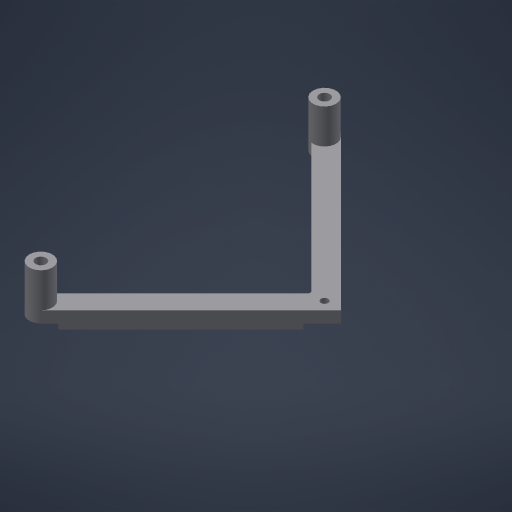
# Autodesk Inventor part: WIDE SCREEN HOLDER 2SCREEN
Saved by Autodesk Inventor 2023.3 (Build 273359000, 359)
## iProperties
RuleStatus: InUse
Created: 2023-07-19
Material: Generic
Catalog Web Link: https://www.janelia.org/
Vendor: HHMI: JRC - jET
Document SubType Name: Modeling
Designer: jagers
Density: 1 g/cm^3
Appearance: Default
Part Number: WIDE SCREEN HOLDER 2SCREEN
AfterDocSave0: file://Part Number Cleaner
DESIGN DEPARTMENT: HHMI: JRC - jET
ALTERED ITEM PART NUMBER: N/A
ALTERED ITEM VENDOR: N/A
ALTERED ITEM DESCRIPTION: N/A
Title: Standard
Author: jagers
Revision Number: 0
Autodesk Inventor part; units mm, degrees
ref_plane "YZ Plane" through (0, 0, 0) normal (1, 0, 0) x (0, 1, 0)
ref_plane "XZ Plane" through (0, 0, 0) normal (0, 1, 0) x (-1, 0, 0)
sketch "Sketch1" plane through (0, 0, 0) normal (0, 1, 0) x (-1, 0, 0)
  line L0 (-41.3092, 0) -> (0, 41.3092)
  circle A0 centre (-36.8191, 0) radius 1.016
  arc A1 (-32.8821, 0) -> (-34.0352, 2.7839) centre (-36.8191, 0) ccw
  line L1 (0, 41.3092) -> (2.2451, 39.0641)
  arc A2 (0, 36.8191) -> (0, 41.3092) centre (2.2451, 39.0641) ccw
  circle A3 centre (2.2451, 39.0641) radius 1.4732
  line L2 (0, 36.8191) -> (-34.0352, 2.7839)
  line L3 (0, 0) -> (-14.0183, 0)
  line L4 (-41.3092, 0) -> (0, -41.3092)
  circle A4 centre (-36.8191, 0) radius 1.016
  arc A5 (-34.0352, -2.7839) -> (-32.8821, 0) centre (-36.8191, 0) ccw
  line L5 (0, -41.3092) -> (2.2451, -39.0641)
  arc A6 (0, -41.3092) -> (0, -36.8191) centre (2.2451, -39.0641) ccw
  circle A7 centre (2.2451, -39.0641) radius 1.4732
  line L6 (0, -36.8191) -> (-34.0352, -2.7839)
  dimension "d0" = 3.175
  dimension "d1" = 58.42
  dimension "d2" = 45
  dimension "d3" = 2.9464
  dimension "d4" = 3.175
  dimension "d5" = 3.937
  dimension "d6" = 2.032
  dimension "d7" = 45
  constraints: 14 end point, 10 point on circle, 8 centre point, 6 coincident, 6 symmetric about line, 3 horizontal alignment, 1 horizontal, 1 parallel, 1 perpendicular, 1 vertical alignment, 4 other
  measures "d0" distance between parallel lines of L0 L2
  measures "d1" distance from line of L0.start L1
  measures "d3" diameter of A3
  measures "d4" radius of A2
  measures "d5" radius of A1
  measures "d6" diameter of A0
  measures "d7" angle of L2 L3
extrude "Extrusion1" add sketch "Sketch1" along normal blind 3.175
sketch "Sketch2" plane through (0, 3.175, 0) normal (0, 1, 0) x (1, 0, 0)
  circle A0 centre (-2.2451, -39.0641) radius 1.4732 projected
  circle A1 centre (-2.2451, -39.0641) radius 3.175
  circle A2 centre (-2.2451, 39.0641) radius 1.4732 projected
  circle A3 centre (-2.2451, 39.0641) radius 3.175
  point P0 (0, 0)
  dimension "d10" = 6.35
  dimension "d11" = 6.35
  constraints: 2 centre point, 2 coincident
  measures "d10" diameter of A1
  measures "d11" diameter of A3
extrude "Extrusion2" add sketch "Sketch2" along normal blind 9.525
chamfer "Chamfer1" distance 1.27 angle 45 2 edges at (-0.7719, 0, 39.0641) (-0.7719, 0, -39.0641)
sketch "Sketch3" plane through (0, 3.175, 0) normal (0, 1, 0) x (1, 0, 0)
  arc A0 (0, -36.8191) -> (0, -41.3092) centre (-2.2451, -39.0641) ccw projected
  line L0 (34.0352, -2.7839) -> (0, -36.8191) projected
  arc A1 (34.0352, 2.7839) -> (34.0352, -2.7839) centre (36.8191, 0) ccw projected
  line L1 (0, 36.8191) -> (34.0352, 2.7839) projected
  arc A2 (0, 41.3092) -> (0, 36.8191) centre (-2.2451, 39.0641) ccw projected
  line L2 (-2.6941, -35.921) -> (32.896, -0.331)
  arc A3 (34.0352, 2.7839) -> (34.0352, -2.7839) centre (36.8191, 0) ccw projected
  line L3 (32.896, 0.331) -> (-2.6941, 35.921)
  point P0 (0, 0)
  dimension "d17" = 2.54
  dimension "d18" = 2.54
  constraints: 4 end point, 4 point on circle, 1 parallel
  measures "d17" distance between parallel lines of L3 L1
  measures "d18" distance between parallel lines of L0 L2
ref_plane "Work Plane1" through (0, -3.81, 0) normal (0, 1, 0) x (1, 0, 0)
extrude "Extrusion3" add sketch "Sketch3" against normal up to surface (3.175 mm away)
sketch "Sketch4" plane through (0, 0, 0) normal (0, -1, 0) x (1, 0, 0)
  line L0 (0, -36.8191) -> (34.0352, -2.7839) projected
  line L1 (0, 36.8191) -> (34.0352, 2.7839) projected
  line L2 (-2.6941, -35.921) -> (32.896, -0.331) projected
  line L3 (-1.6524, -34.8793) -> (32.0954, -1.1315)
  line L4 (32.0954, -1.1315) -> (33.7478, -2.7839)
  line L5 (33.7478, -2.7839) -> (0, -36.5317)
  line L6 (0, -36.5317) -> (-1.6524, -34.8793)
  line L7 (0, 0) -> (11.5163, 0)
  line L8 (-1.6524, 34.8793) -> (32.0954, 1.1315)
  line L9 (32.0954, 1.1315) -> (33.7478, 2.7839)
  line L10 (33.7478, 2.7839) -> (0, 36.5317)
  line L11 (0, 36.5317) -> (-1.6524, 34.8793)
  dimension "d22" = 0.2032
  dimension "d23" = 0.2032
  dimension "d24" = 0.2032
  constraints: 18 end point, 4 symmetric about line, 2 parallel, 2 point on line, 1 horizontal, 1 perpendicular
  measures "d22" distance between parallel lines of L0 L5
  measures "d23" distance from line of L0.end L4
  measures "d24" distance from line of L0.start L6
extrude "Extrusion4" add sketch "Sketch4" along normal up to surface (3.81 mm away)
chamfer "Chamfer2" distance 2.3368 angle 45 4 edges at (-1.6524, -1.905, -34.8793) (-1.6524, -1.905, 34.8793) (32.0954, -1.905, 1.1315) (32.0954, -1.905, -1.1315)
body "Solid1"
